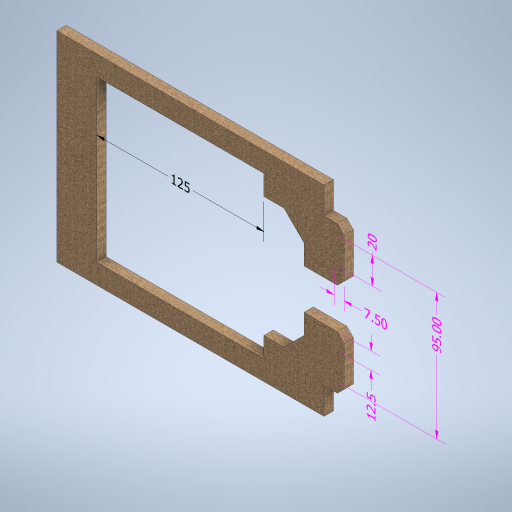
# Autodesk Inventor part: Marco
Saved by Autodesk Inventor 2023.1 (Build 271208000, 208)
## iProperties
Created: 2022-10-28
Part Number: Marco
Material: MDF Medium Density Fiberboard
Document SubType Name: Modeling
Designer: Daniel Peña
Density: 0.8 g/cm^3
Appearance: Cardboard - Corrugated
Author: Daniel Peña
Autodesk Inventor part; units mm, degrees
ref_plane "YZ Plane" through (0, 0, 0) normal (1, 0, 0) x (0, 1, 0)
ref_plane "XZ Plane" through (0, 0, 0) normal (0, 1, 0) x (-1, 0, 0)
ref_plane "XY Plane" through (0, 0, 0) normal (0, 0, 1) x (1, 0, 0)
sketch "Sketch1" plane through (0, 0, 0) normal (0, 0, 1) x (1, 0, 0)
  line L0 (-100, -75) -> (100, -75) projected
  line L1 (100, -75) -> (100, 75) projected
  line L2 (100, 75) -> (-100, 75) projected
  line L3 (-100, 75) -> (-100, -75) projected
  line L4 (-70, -60) -> (55, -60)
  line L5 (55, 60) -> (-70, 60)
  line L6 (-70, 60) -> (-70, 15)
  line L7 (-70, -15) -> (-70, -60)
  line L8 (151.2343, 15) -> (1.2343, 15) projected
  line L9 (1.2343, -15) -> (151.2343, -15) projected
  line L10 (85, -30) -> (85, -15)
  line L11 (85, 15) -> (85, 30)
  line L12 (-100, 75) -> (100, 75)
  line L13 (100, -75) -> (-100, -75)
  line L14 (-100, -75) -> (-100, 75)
  line L15 (100, -15) -> (85, -15)
  line L16 (100, 15) -> (85, 15)
  line L17 (-100, 0) -> (100, 0) construction
  line L18 (70, 45) -> (70, -45) projected
  line L19 (70, -45) -> (-70, -45) projected
  line L20 (-70, -45) -> (-70, 45) projected
  line L21 (-70, 45) -> (70, 45) projected
  line L22 (-70, 15) -> (-70, -15)
  line L23 (85, -30) -> (70, -45)
  line L24 (70, -45) -> (55, -45)
  line L25 (55, -45) -> (55, -60)
  line L26 (85, 30) -> (70, 45)
  line L27 (70, 45) -> (55, 45)
  line L28 (55, 45) -> (55, 60)
  line L29 (100, -55) -> (110, -55)
  line L30 (115, -50) -> (115, -20)
  line L31 (110, -55) -> (115, -50)
  line L32 (110, -15) -> (100, -15)
  line L33 (115, -20) -> (110, -15)
  line L34 (100, 55) -> (110, 55)
  line L35 (115, 50) -> (115, 20)
  line L36 (110, 55) -> (115, 50)
  line L37 (110, 15) -> (100, 15)
  line L38 (115, 20) -> (110, 15)
  line L39 (100, 55) -> (100, 75)
  line L40 (100, -55) -> (100, -75)
  point P0 (0, 0)
  point P1 (85, -60)
  point P2 (85, 60)
  point P3 (100, 15)
  point P4 (100, -15)
  point P5 (-70, 15)
  point P6 (85, -22.5)
  point P7 (70, 15)
  point P8 (70, -15)
  point P9 (115, -55)
  point P10 (115, -15)
  point P11 (100, -15)
  point P12 (100, 55)
  point P13 (100, 15)
  dimension "d3" = 15
  dimension "d4" = 15
  dimension "d5" = 30
  dimension "d13" = 30
  dimension "d17" = 5
  dimension "d18" = 5
  dimension "d33" = 15
  dimension "d35" = 5
  dimension "d36" = 5
  constraints: 62 end point, 12 point on line, 5 collinear, 3 midpoint, 3 symmetric about line, 2 horizontal, 1 parallel, 1 perpendicular, 3 other
  measures "d3" distance between parallel lines of L1 L11
  measures "d4" distance between parallel lines of L12 L5
  measures "d5" distance between parallel lines of L3 L6
  measures "d13" distance of L5.start point (85, 60)
  measures "d17" distance of L29.end point (115, -55)
  measures "d18" distance of L30.start point (115, -55)
  measures "d33" distance of point (115, -15) L32.end
  measures "d35" distance of L30.end point (115, -15)
  measures "d36" distance of L32.start point (115, -15)
extrude "Extrusion1" add sketch "Sketch1" along normal blind 7 contours L3 L2 L1 L8 L11 L26 L21 L28 L5 L6 L20 L7 L4 L25 L19 L23 L10 L9 L0 | L1 L9 L33 L30 L31 L29 | L34 L36 L35 L38 L8 L1
sketch "Sketch2" plane through (0, 0, 7) normal (0, 0, 1) x (1, 0, 0)
  line L0 (-70, -60) -> (-70, 60) construction
  line L1 (-70, 0) -> (130.7679, 0) construction
  line L2 (115, -50) -> (115, -20) construction
  line L3 (-100, -55) -> (110, -55) construction
  line L4 (100, -15) -> (85, -15) construction
  point P0 (0, 0)
  point P1 (107.5, -75)
  point P2 (107.5, -95)
  point P3 (107.5, 75)
  point P4 (107.5, 95)
  point P5 (115, -20)
  point P6 (-100, -75)
  point P7 (110, -15)
  dimension "d21" = 7.5
  dimension "d24" = 7.5
  dimension "d32" = 20
  dimension "d73" = 150
  constraints: 2 end point, 2 symmetric about line, 1 horizontal, 1 midpoint
  measures "d21" distance from line of L2 point (107.5, -95)
  measures "d24" distance from line of L2 point (107.5, -75)
  measures "d32" distance of point (107.5, -95) point (107.5, -75)
  measures "d73" distance of point (107.5, -75) point (107.5, 75)
hole "Hole1" at (107.5, -75, 7) at (107.5, -95, 7) at (107.5, 75, 7) at (107.5, 95, 7) direction (0, 0, -1) diameter 4 end through all
body "Solid1"
